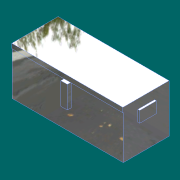
# Autodesk Inventor part: Aluminum tool box
Saved by Autodesk Inventor 2017 (Build 210142000, 142)
## iProperties
Created: 2018-01-23
Part Number: Aluminum tool box
Material: Aluminum 6061
Document SubType Name: Modeling
Designer: Graeme_Van_Dongen
Density: 2.7 g/cm^3
Appearance: Aluminum - Flat
Author: Graeme_Van_Dongen
Autodesk Inventor part; units mm, degrees
ref_plane "YZ Plane" through (0, 0, 0) normal (1, 0, 0) x (0, 1, 0)
ref_plane "XZ Plane" through (0, 0, 0) normal (0, 1, 0) x (-1, 0, 0)
sketch "Sketch1" plane through (0, 0, 0) normal (0, 1, 0) x (-1, 0, 0)
  line L0 (381, 157.1625) -> (-381, 157.1625)
  line L1 (-381, 157.1625) -> (-381, -157.1625)
  line L2 (-381, -157.1625) -> (381, -157.1625)
  line L3 (381, -157.1625) -> (381, 157.1625)
  line L4 (381, 157.1625) -> (-381, -157.1625) construction
  line L5 (-381, 157.1625) -> (381, -157.1625) construction
  point P0 (0, 0)
  dimension "d0" = 762
  dimension "d1" = 314.325
  constraints: 12 end point, 2 midpoint, 2 parallel, 1 horizontal, 1 perpendicular
  measures "d0" distance of L2.end L1.end
  measures "d1" distance of L1.end L0.end
extrude "Extrusion1" add sketch "Sketch1" along normal blind 330.2
sketch "Sketch2" plane through (0, 330.2, 0) normal (0, 1, 0) x (1, 0, 0)
  line L0 (-381, 157.1625) -> (-381, -157.1625) projected
  line L1 (381, 157.1625) -> (-381, 157.1625) projected
  line L2 (381, -157.1625) -> (381, 157.1625) projected
  line L3 (-381, -157.1625) -> (-381, -160.3375)
  line L4 (-381, -160.3375) -> (381, -160.3375)
  line L5 (381, -160.3375) -> (381, -157.1625)
  point P0 (0, 0)
  dimension "d4" = 3.175
  constraints: 6 end point, 2 perpendicular, 1 vertical
  measures "d4" distance of L0.end L3.end
extrude "Extrusion2" add sketch "Sketch2" against normal blind 31.75
sketch "Sketch3" plane through (-381, 0, 157.1625) normal (0, 0, 1) x (1, 0, 0)
  line L0 (358.775, 146.05) -> (403.225, 146.05)
  line L1 (403.225, 146.05) -> (403.225, 298.45)
  line L2 (403.225, 298.45) -> (358.775, 298.45)
  line L3 (358.775, 298.45) -> (358.775, 146.05)
  line L4 (762, 298.45) -> (0, 298.45) construction
  point P0 (381, 0)
  point P1 (381, 146.05)
  dimension "d7" = 44.45
  dimension "d8" = 146.05
  constraints: 8 end point, 2 parallel, 1 collinear, 1 horizontal, 1 midpoint, 1 perpendicular, 1 vertical alignment
  measures "d7" distance of L2.end L1.end
  measures "d8" distance from line of L0 point (381, 0)
extrude "Extrusion3" add sketch "Sketch3" along normal blind 25.4
sketch "Sketch4" plane through (381, 0, 157.1625) normal (1, 0, 0) x (0, 0, -1)
  line L0 (100.0125, 190.5) -> (214.3125, 190.5)
  line L1 (214.3125, 190.5) -> (214.3125, 266.7)
  line L2 (214.3125, 266.7) -> (100.0125, 266.7)
  line L3 (100.0125, 266.7) -> (100.0125, 190.5)
  point P0 (157.1625, 0)
  point P1 (157.1625, 190.5)
  dimension "d11" = 114.3
  dimension "d12" = 190.5
  dimension "d13" = 76.2
  constraints: 8 end point, 2 parallel, 1 horizontal, 1 midpoint, 1 perpendicular, 1 vertical alignment
  measures "d11" distance of L2.end L1.end
  measures "d12" distance from line of point (157.162, 0) L0
  measures "d13" distance of L0.end L1.end
extrude "Extrusion4" add sketch "Sketch4" along normal blind 12.7
ref_plane "Work Plane1" through (311.15, 0, 157.1625) normal (1, 0, 0) x (0, 0, -1)
sketch "Sketch5" plane through (311.15, 0, 157.1625) normal (1, 0, 0) x (0, 0, -1)
  line L0 (314.325, 0) -> (314.325, 330.2) construction
  line L1 (0, 298.45) -> (-3.175, 298.45) construction
  circle A0 centre (322.2625, 298.45) radius 7.9375
  point P0 (157.1625, 0)
  dimension "d17" = 15.875
  constraints: 1 centre point, 1 point on line, 1 tangent
  measures "d17" diameter of A0
extrude "Extrusion5" add sketch "Sketch5" against normal blind 101.6
mirror "Mirror1" about plane through (0, 0, 0) normal (1, 0, 0) of "Extrusion5", "Extrusion4"
body "Solid1"
